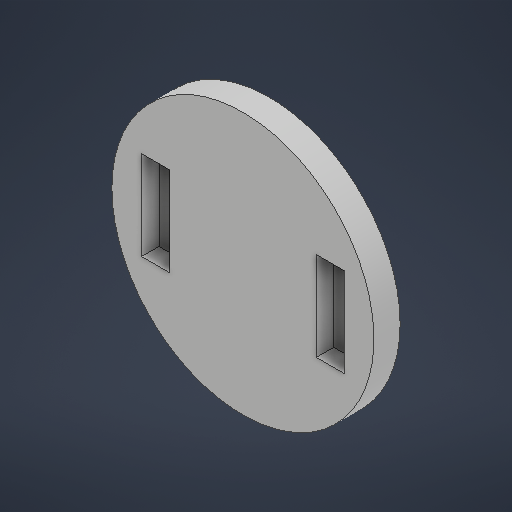
# Autodesk Inventor part: Tag
Saved by Autodesk Inventor 2026.1 (Build 301233020, 233B)
## iProperties
Created: 2026-04-07
Part Number: Tag
Material: Generic
Document SubType Name: Modeling
Designer: Bahaa
Mass: 1.89954 g
Surface Area: 18.1874 cm^2
Volume: 1.89954 cm^3
Density: 1 g/cm^3
Appearance: Default
Author: Bahaa
Mass: 1.91341 g
Surface Area: 18.3174 cm^2
Volume: 1.91341 cm^3
Autodesk Inventor part; units mm, degrees
ref_plane "YZ Plane" through (0, 0, 0) normal (1, 0, 0) x (0, 1, 0)
ref_plane "XZ Plane" through (0, 0, 0) normal (0, 1, 0) x (-1, 0, 0)
ref_plane "XY Plane" through (0, 0, 0) normal (0, 0, 1) x (1, 0, 0)
sketch "Sketch1" plane through (0, 0, 0) normal (0, 1, 0) x (-1, 0, 0)
  circle A0 centre (0, 0) radius 15
  dimension "d0" = 30
  constraints: 1 centre point, 1 coincident
  measures "d0" diameter of A0
extrude "Extrusion1" add sketch "Sketch1" against normal blind 2.8
sketch "Sketch2" plane through (0, 0, 0) normal (0, 1, 0) x (1, 0, 0)
  line L0 (7.5, -7.5) -> (-7.5, -7.5)
  line L1 (-7.5, -7.5) -> (-7.5, 7.5)
  line L2 (-7.5, 7.5) -> (7.5, 7.5)
  line L3 (7.5, 7.5) -> (7.5, -7.5)
  line L4 (7.5, -7.5) -> (-7.5, 7.5) construction
  line L5 (-7.5, -7.5) -> (7.5, 7.5) construction
  circle A0 centre (0, 0) radius 12
  circle A1 centre (0, 0) radius 15 projected
  dimension "d3" = 15
  dimension "d4" = 15
  dimension "d13" = 3
  constraints: 12 end point, 3 coincident, 2 midpoint, 2 parallel, 1 centre point, 1 horizontal, 1 perpendicular, 2 other
  measures "d3" distance of L1.end L2.end
  measures "d4" distance of L0.end L1.end
  measures "d13" radial gap between concentric circles of A1 A0
extrude "Extrusion2" add sketch "Sketch2" along normal blind 0.2 contours A1
sketch "Sketch3" plane through (0, -2.8, 0) normal (0, -1, 0) x (1, 0, 0)
  line L0 (10, 0) -> (-10, 0) construction
  line L1 (-11.6, -5.1) -> (-8.4, -5.1)
  line L2 (-8.4, -5.1) -> (-8.4, 5.1)
  line L3 (-8.4, 5.1) -> (-11.6, 5.1)
  line L4 (-11.6, 5.1) -> (-11.6, -5.1)
  line L5 (-11.6, -5.1) -> (-8.4, 5.1) construction
  line L6 (-8.4, -5.1) -> (-11.6, 5.1) construction
  line L7 (0, -15) -> (0, 15) construction
  circle A0 centre (0, 0) radius 15 construction
  line L8 (11.6, -5.1) -> (8.4, -5.1)
  line L9 (8.4, -5.1) -> (8.4, 5.1)
  line L10 (8.4, 5.1) -> (11.6, 5.1)
  line L11 (11.6, 5.1) -> (11.6, -5.1)
  line L12 (11.6, -5.1) -> (8.4, 5.1) construction
  line L13 (8.4, -5.1) -> (11.6, 5.1) construction
  dimension "d14" = 20
  dimension "d15" = 3.2
  dimension "d16" = 10.2
  constraints: 28 end point, 4 midpoint, 4 symmetric about line, 2 horizontal, 2 parallel, 1 perpendicular, 1 point on circle, 1 vertical
  measures "d14" distance of L0.start L0.end
  measures "d15" distance of L3.end L2.end
  measures "d16" distance of L2.end L1.end
extrude "Extrusion3" cut sketch "Sketch3" against normal blind 2
extrude "Extrusion4" [suppressed]
extrude "Extrusion5" [suppressed]
body "Solid1"
